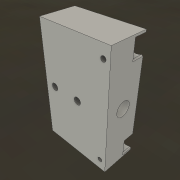
# Autodesk Inventor part: MotorMountLeft
Saved by Autodesk Inventor 2019.3 (Build 233278000, 278)
## iProperties
Created: 2019-01-26
Part Number: MotorMountLeft
Material: Generic
Document SubType Name: Modeling
Designer: mark
Density: 1 g/cm^3
Appearance: Default
Mass: 337.734 g
Surface Area: 418.977 cm^2
Volume: 337.734 cm^3
Author: mark
Autodesk Inventor part; units mm, degrees
ref_plane "YZ Plane" through (0, 0, 0) normal (1, 0, 0) x (0, 1, 0)
ref_plane "XZ Plane" through (0, 0, 0) normal (0, 1, 0) x (-1, 0, 0)
ref_plane "XY Plane" through (0, 0, 0) normal (0, 0, 1) x (1, 0, 0)
sketch "Sketch1" plane through (0, 0, 0) normal (0, 0, 1) x (1, 0, 0)
  line L0 (0, 0) -> (76.2, 0)
  line L1 (76.2, 0) -> (76.2, 125.8)
  line L2 (76.2, 125.8) -> (0, 125.8)
  line L3 (0, 125.8) -> (0, 0)
  circle A0 centre (12, 62.9) radius 4
  circle A1 centre (42, 62.9) radius 4
  dimension "d0" = 76.2
  dimension "d1" = 125.8
  dimension "d2" = 8
  dimension "d3" = 8
  dimension "d4" = 12
  dimension "d5" = 42
  dimension "d6" = 62.9
  dimension "d7" = 62.9
  constraints: 8 end point, 2 centre point, 2 perpendicular, 1 horizontal
  measures "d0" distance of L2.end L1.end
  measures "d1" distance between parallel lines of L0 L2
  measures "d2" diameter of A0
  measures "d3" diameter of A1
  measures "d4" distance from line of L3 A0.centre
  measures "d5" distance from line of L3 A1.centre
  measures "d6" distance from line of L0 A1.centre
  measures "d7" distance from line of L0 A0.centre
extrude "Extrusion1" add sketch "Sketch1" along normal blind 38.2 contours L3 L2 L1 L0 | A0 | A1
sketch "Sketch2" plane through (0, 0, 38.2) normal (0, 0, 1) x (1, 0, 0)
  line L0 (0, 0) -> (76.2, 0)
  line L1 (76.2, 0) -> (76.2, 125.8)
  line L2 (76.2, 125.8) -> (0, 125.8)
  line L3 (0, 125.8) -> (0, 0)
  circle A0 centre (12, 62.9) radius 4
  circle A1 centre (42, 62.9) radius 4
  dimension "d17" = 76.2
  dimension "d16" = 125.8
  dimension "d13" = 8
  dimension "d10" = 8
  dimension "d15" = 12
  dimension "d12" = 42
  dimension "d11" = 62.9
  dimension "d14" = 62.9
  constraints: 8 end point, 2 centre point, 2 perpendicular, 1 horizontal
  measures "d17" distance of L2.end L1.end
  measures "d16" distance between parallel lines of L0 L2
  measures "d13" diameter of A0
  measures "d10" diameter of A1
  measures "d15" distance from line of L3 A0.centre
  measures "d12" distance from line of L3 A1.centre
  measures "d11" distance from line of L0 A1.centre
  measures "d14" distance from line of L0 A0.centre
extrude "Extrusion2" cut sketch "Sketch2" against normal blind 19.1 contours A0 | A1
sketch "Sketch3" plane through (0, 0, 0) normal (-1, 0, 0) x (0, 0, 1)
  circle A0 centre (19.1, 62.9) radius 8
  line L0 (38.2, 125.8) -> (38.2, 0) projected
  line L1 (0, 0) -> (38.2, 0) projected
  dimension "d21" = 16
  dimension "d22" = 19.1
  dimension "d23" = 62.9
  constraints: 1 centre point
  measures "d21" diameter of A0
  measures "d22" distance from line of L0 A0.centre
  measures "d23" distance from line of L1 A0.centre
extrude "Extrusion3" cut sketch "Sketch3" against normal up to next
thread "Thread1" size "M8x1.25" class "6H" standard "ANSI Metric M Profile" full length
thread "Thread2" size "M8x1.25" class "6H" standard "ANSI Metric M Profile" full length
sketch "Sketch7" plane through (76.2, 107.525, 0) normal (0, 0, -1) x (-1, 0, 0)
  circle A0 centre (6.335, -95.665) radius 2.5
  circle A1 centre (6.335, 6.335) radius 2.5
  line L0 (0, -89.33) -> (76.2, -89.33) projected
  line L1 (0, -107.525) -> (0, 18.275) projected
  line L2 (0, 18.275) -> (76.2, 18.275) projected
  point P0 (76.2, -107.525)
  dimension "d92" = 5
  dimension "d93" = 5
  dimension "d104" = 102
  dimension "d129" = 6.335
  dimension "d130" = 11.94
  dimension "d131" = 6.335
  constraints: 2 centre point
  measures "d92" diameter of A0
  measures "d93" diameter of A1
  measures "d104" distance of A0.centre A1.centre
  measures "d129" distance from line of L1 A1.centre
  measures "d130" distance from line of L2 A1.centre
  measures "d131" distance from line of L1 A0.centre
extrude "Extrusion7" cut sketch "Sketch7" against normal up to next
thread "Thread11" size "M5x0.8" class "6H" standard "ANSI Metric M Profile" full length
thread "Thread12" size "M5x0.8" class "6H" standard "ANSI Metric M Profile" full length
sketch "Sketch8" plane through (0, 0, 0) normal (0, 0, -1) x (-1, 0, 0)
  circle A0 centre (-8, 45.485) radius 4
  circle A1 centre (-8, 80.235) radius 4
  circle A2 centre (-68.2, 45.485) radius 4
  circle A3 centre (-68.2, 80.235) radius 4
  line L0 (0, 125.8) -> (0, 0) projected
  line L1 (-76.2, 0) -> (-76.2, 125.8) projected
  line L2 (-76.2, 18.195) -> (0, 18.195) projected
  line L3 (0, 107.525) -> (-76.2, 107.525) projected
  dimension "d106" = 8
  dimension "d107" = 8
  dimension "d108" = 8
  dimension "d109" = 8
  dimension "d110" = 8
  dimension "d111" = 8
  dimension "d112" = 8
  dimension "d113" = 8
  dimension "d114" = 34.75
  dimension "d115" = 34.75
  dimension "d116" = 27.29
  dimension "d117" = 27.29
  dimension "d118" = 89.33
  constraints: 4 centre point
  measures "d106" diameter of A0
  measures "d107" diameter of A1
  measures "d108" diameter of A3
  measures "d109" diameter of A2
  measures "d110" distance from line of L0 A0.centre
  measures "d111" distance from line of L0 A1.centre
  measures "d112" distance from line of L1 A2.centre
  measures "d113" distance from line of L1 A3.centre
  measures "d114" distance of A1.centre A0.centre
  measures "d115" distance of A3.centre A2.centre
  measures "d116" distance from line of L2 A0.centre
  measures "d117" distance from line of L2 A2.centre
  measures "d118" distance between parallel lines of L3 L2
extrude "Extrusion8" cut sketch "Sketch8" against normal blind 20 contours A0 | A1 | A2 | A3
thread "Thread13" size "M8x1.25" class "6H" standard "ANSI Metric M Profile" full length
thread "Thread14" size "M8x1.25" class "6H" standard "ANSI Metric M Profile" full length
thread "Thread15" size "M8x1.25" class "6H" standard "ANSI Metric M Profile" full length
thread "Thread16" size "M8x1.25" class "6H" standard "ANSI Metric M Profile" full length
sketch "Sketch9" plane through (0, 0, 0) normal (0, 0, -1) x (-1, 0, 0)
  circle A0 centre (-69.865, 113.86) radius 10
  circle A1 centre (-69.865, 11.86) radius 10
  circle A2 centre (-69.865, 113.86) radius 2.5 projected
  circle A3 centre (-69.865, 11.86) radius 2.5 projected
  point P0 (0, 0)
  dimension "d132" = 20
  dimension "d133" = 20
  constraints: 2 centre point, 2 coincident
  measures "d132" diameter of A0
  measures "d133" diameter of A1
extrude "Extrusion9" cut sketch "Sketch9" against normal blind 12.67
chamfer "Chamfer2" distance 2 angle 45 4 edges at (76.2, 121.5974, 6.335) (76.2, 106.1226, 6.335) (76.2, 4.1226, 6.335) (76.2, 19.5974, 6.335)
body "Solid1"
